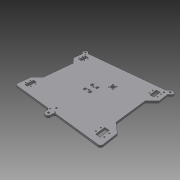
# Autodesk Inventor part: y_carriage_v2
Saved by Autodesk Inventor 2014 (Build 180170000, 170)
## iProperties
Created: 2013-12-03
Part Number: y_carriage_v2
Material: Generic
Document SubType Name: Modeling
Designer: buben
Density: 1 g/cm^3
Appearance: Default
Author: buben
Subject: Laser Cutted
Autodesk Inventor part; units mm, degrees
ref_plane "YZ Plane" through (0, 0, 0) normal (1, 0, 0) x (0, 1, 0)
ref_plane "XZ Plane" through (0, 0, 0) normal (0, 1, 0) x (-1, 0, 0)
ref_plane "XY Plane" through (0, 0, 0) normal (0, 0, 1) x (1, 0, 0)
sketch "Sketch1" plane through (0, 0, 0) normal (0, 0, 1) x (1, 0, 0)
  line L0 (267.8905, 0) -> (267.8905, 212.6863)
  line L1 (256.5768, 224) -> (11.3137, 224)
  line L2 (0, 212.6863) -> (0, 0)
  line L3 (0, 224) -> (267.8905, 224) construction
  line L4 (267.8905, 224) -> (133.9453, -8) construction
  line L5 (133.9453, -8) -> (0, 224) construction
  circle A0 centre (0, 224) radius 2.75
  circle A1 centre (133.9453, -8) radius 2.75
  circle A2 centre (267.8905, 224) radius 2.75
  circle A3 centre (0, 224) radius 5 construction
  circle A4 centre (267.8905, 224) radius 5 construction
  circle A5 centre (133.9453, -8) radius 5 construction
  line L6 (-2.8284, 232.4853) -> (-8.4853, 226.8284)
  line L7 (-8.4853, 226.8284) -> (-8.4853, 221.1716)
  line L8 (-2.8284, 232.4853) -> (2.8284, 232.4853)
  line L9 (2.8284, 232.4853) -> (11.3137, 224)
  line L10 (-8.4853, 221.1716) -> (0, 212.6863)
  line L11 (125.9453, 0) -> (125.9453, -12)
  line L12 (125.9453, -12) -> (129.9453, -16)
  line L13 (129.9453, -16) -> (137.9453, -16)
  line L14 (137.9453, -16) -> (141.9453, -12)
  line L15 (141.9453, -12) -> (141.9453, 0)
  line L16 (267.8905, 212.6863) -> (276.3758, 221.1716)
  line L17 (276.3758, 221.1716) -> (276.3758, 226.8284)
  line L18 (276.3758, 226.8284) -> (270.719, 232.4853)
  line L19 (270.719, 232.4853) -> (265.0621, 232.4853)
  line L20 (265.0621, 232.4853) -> (256.5768, 224)
  line L21 (0, 0) -> (125.9453, 0)
  line L22 (141.9453, 0) -> (267.8905, 0)
  dimension "d0" = 5.5
  dimension "d1" = 5.5
  dimension "d2" = 5.5
  dimension "d3" = 10
  dimension "d4" = 10
  dimension "d5" = 10
  dimension "d6" = 232
  dimension "d7" = 45
  dimension "d8" = 8
  dimension "d9" = 4
  dimension "d10" = 8
  dimension "d11" = 8
  dimension "d12" = 4
  dimension "d13" = 45
  dimension "d15" = 12
  dimension "d17" = 45
  dimension "d18" = 8
  dimension "d19" = 4
  dimension "d20" = 8
  dimension "d45" = 45
  dimension "d46" = 8
  dimension "d47" = 45
  dimension "d48" = 8
  dimension "d49" = 8
  dimension "d50" = 8
  constraints: 46 end point, 10 perpendicular, 7 coincident, 7 equal length, 6 centre point, 6 parallel, 2 collinear, 2 horizontal
  measures "d0" diameter of A1
  measures "d1" diameter of A0
  measures "d2" diameter of A2
  measures "d3" diameter of A4
  measures "d4" diameter of A5
  measures "d5" diameter of A3
  measures "d6" distance from line of L3 L4.end
  measures "d7" angle of L7 L6
  measures "d8" distance from line of L3.start L6
  measures "d9" distance from line of L6.end L10
  measures "d10" distance of L6.start L6.end
  measures "d11" distance of L12.end L13.end
  measures "d12" horizontal distance of L11.end L12.end
  measures "d13" angle of L13 L12
  measures "d15" distance of L14.end L15.end
  measures "d17" angle of L17 L18
  measures "d18" distance of L17.end L18.end
  measures "d19" distance from line of L18.end L20
  measures "d20" distance from line of L18 L3.end
  measures "d45" angle of L9 L1
  measures "d46" distance from line of L10 L3.start
  measures "d47" angle of L20 L1
  measures "d48" distance from line of L20 L3.end
  measures "d49" distance from line of L13 L4.end
  measures "d50" distance from line of L11 L4.end
extrude "Extrusion2" add sketch "Sketch1" along normal blind 6
sketch "Sketch3" plane through (0, 0, 6) normal (0, 0, 1) x (1, 0, 0)
  line L0 (0, 212.6863) -> (0, 0) projected
  line L1 (0, 0) -> (125.9453, 0) projected
  line L2 (267.8905, 0) -> (267.8905, 212.6863) projected
  line L3 (256.5768, 224) -> (11.3137, 224) projected
  line L4 (16.4453, 209) -> (25.4453, 209)
  line L5 (26.4453, 208) -> (26.4453, 185)
  line L6 (25.4453, 184) -> (16.4453, 184)
  line L7 (15.4453, 185) -> (15.4453, 208)
  arc A0 (16.4453, 209) -> (15.4453, 208) centre (16.4453, 208) ccw
  arc A1 (15.4453, 185) -> (16.4453, 184) centre (16.4453, 185) ccw
  arc A2 (25.4453, 184) -> (26.4453, 185) centre (25.4453, 185) ccw
  arc A3 (26.4453, 208) -> (25.4453, 209) centre (25.4453, 208) ccw
  line L8 (242.4453, 209) -> (251.4453, 209)
  line L9 (252.4453, 208) -> (252.4453, 185)
  line L10 (251.4453, 184) -> (242.4453, 184)
  line L11 (241.4453, 185) -> (241.4453, 208)
  arc A4 (242.4453, 209) -> (241.4453, 208) centre (242.4453, 208) ccw
  arc A5 (241.4453, 185) -> (242.4453, 184) centre (242.4453, 185) ccw
  arc A6 (251.4453, 184) -> (252.4453, 185) centre (251.4453, 185) ccw
  arc A7 (252.4453, 208) -> (251.4453, 209) centre (251.4453, 208) ccw
  line L12 (242.4453, 40) -> (251.4453, 40)
  line L13 (252.4453, 39) -> (252.4453, 16)
  line L14 (251.4453, 15) -> (242.4453, 15)
  line L15 (241.4453, 16) -> (241.4453, 39)
  arc A8 (242.4453, 40) -> (241.4453, 39) centre (242.4453, 39) ccw
  arc A9 (241.4453, 16) -> (242.4453, 15) centre (242.4453, 16) ccw
  arc A10 (251.4453, 15) -> (252.4453, 16) centre (251.4453, 16) ccw
  arc A11 (252.4453, 39) -> (251.4453, 40) centre (251.4453, 39) ccw
  line L16 (16.4453, 40) -> (25.4453, 40)
  line L17 (26.4453, 39) -> (26.4453, 16)
  line L18 (25.4453, 15) -> (16.4453, 15)
  line L19 (15.4453, 16) -> (15.4453, 39)
  arc A12 (16.4453, 40) -> (15.4453, 39) centre (16.4453, 39) ccw
  arc A13 (15.4453, 16) -> (16.4453, 15) centre (16.4453, 16) ccw
  arc A14 (25.4453, 15) -> (26.4453, 16) centre (25.4453, 16) ccw
  arc A15 (26.4453, 39) -> (25.4453, 40) centre (25.4453, 39) ccw
  line L20 (0, 180) -> (20.9453, 159.0547)
  line L21 (20.9453, 159.0547) -> (20.9453, 64.9453)
  line L22 (20.9453, 64.9453) -> (0, 44)
  line L23 (267.8905, 180) -> (246.9453, 159.0547)
  line L24 (246.9453, 159.0547) -> (246.9453, 64.9453)
  line L25 (246.9453, 64.9453) -> (267.8905, 44)
  line L26 (0, 180) -> (0, 44)
  line L27 (267.8905, 180) -> (267.8905, 44)
  line L28 (-8.4853, 226.8284) -> (-8.4853, 221.1716) projected
  line L29 (26.4453, 196.5) -> (241.4453, 196.5) construction
  point P0 (20.9453, 184)
  point P1 (20.9453, 40)
  point P2 (246.9453, 184)
  point P3 (246.9453, 40)
  point P4 (26.4453, 27.5)
  point P5 (241.4453, 27.5)
  point P6 (133.9453, 196.5)
  point P7 (133.9453, 224)
  dimension "d66" = 1
  dimension "d67" = 11
  dimension "d68" = 25
  dimension "d69" = 1
  dimension "d70" = 11
  dimension "d71" = 25
  dimension "d72" = 1
  dimension "d73" = 11
  dimension "d74" = 25
  dimension "d75" = 1
  dimension "d76" = 11
  dimension "d77" = 25
  dimension "d82" = 15
  dimension "d84" = 45
  dimension "d85" = 45
  dimension "d86" = 15
  dimension "d88" = 4
  dimension "d89" = 4
  dimension "d139" = 226
  constraints: 50 end point, 32 point on circle, 32 tangent, 16 centre point, 12 equal radius, 10 midpoint, 9 parallel, 8 perpendicular, 5 vertical alignment, 4 horizontal, 4 horizontal alignment, 4 point on line, 2 collinear
  measures "d66" radius of A0
  measures "d67" distance between parallel lines of L5 L7
  measures "d68" distance between parallel lines of L6 L4
  measures "d69" radius of A4
  measures "d70" distance between parallel lines of L9 L11
  measures "d71" distance between parallel lines of L10 L8
  measures "d72" radius of A8
  measures "d73" distance between parallel lines of L13 L15
  measures "d74" distance between parallel lines of L14 L12
  measures "d75" radius of A12
  measures "d76" distance between parallel lines of L17 L19
  measures "d77" distance between parallel lines of L18 L16
  measures "d82" distance between parallel lines of L3 L4
  measures "d84" angle of L2 L23
  measures "d85" angle of L0 L20
  measures "d86" distance between parallel lines of L1 L18
  measures "d88" distance from line of L22.end L16
  measures "d89" distance from line of L6 L20.start
  measures "d139" distance of point (246.945, 184) point (20.945, 184)
extrude "Extrusion3" cut sketch "Sketch3" against normal blind 6
chamfer "Chamfer1" distance 4 angle 45 4 edges at (0, 0, 3) (125.9453, 0, 3) (141.9453, 0, 3) (267.8905, 0, 3)
sketch "Sketch6" plane through (0, 0, 6) normal (0, 0, 1) x (1, 0, 0)
  line L0 (276.3758, 226.8284) -> (270.719, 232.4853) projected
  line L1 (-2.8284, 232.4853) -> (-8.4853, 226.8284) projected
  line L2 (16.4453, 40) -> (25.4453, 40) projected
  circle A0 centre (267.8905, 224) radius 2.75 projected
  circle A1 centre (133.9453, -8) radius 2.75 projected
  circle A2 centre (0, 224) radius 2.75 projected
  circle A3 centre (9.8995, 214.1005) radius 2.25
  line L3 (-5.6569, 229.6569) -> (9.8995, 214.1005) construction
  circle A4 centre (9.8995, 214.1005) radius 4.5 construction
  circle A5 centre (0, 224) radius 5 construction
  line L4 (11.3137, 224) -> (0, 212.6863) construction
  circle A6 centre (257.991, 214.1005) radius 2.25
  line L5 (273.5474, 229.6569) -> (257.991, 214.1005) construction
  circle A7 centre (133.9453, 12) radius 2.25
  circle A8 centre (125.9453, 2) radius 1.5
  circle A9 centre (141.9453, 2) radius 1.5
  line L6 (133.9453, -8) -> (133.9453, 12) construction
  circle A10 centre (133.9453, 12) radius 4.5 construction
  point P0 (125.9453, -4)
  point P1 (141.9453, -4)
  point P2 (0, 0)
  dimension "d103" = 4.5
  dimension "d105" = 14
  dimension "d106" = 10
  dimension "d107" = 9
  dimension "d108" = 4.5
  dimension "d109" = 14
  dimension "d110" = 4.5
  dimension "d111" = 20
  dimension "d112" = 3
  dimension "d113" = 9
  dimension "d114" = 10
  constraints: 8 centre point, 8 end point, 3 coincident, 3 vertical alignment, 2 midpoint, 2 perpendicular, 2 point on line, 1 equal radius, 1 horizontal alignment
  measures "d103" diameter of A3
  measures "d105" distance of L3.end A2.centre
  measures "d106" diameter of A5
  measures "d107" diameter of A4
  measures "d108" diameter of A6
  measures "d109" distance of L5.end A0.centre
  measures "d110" diameter of A7
  measures "d111" distance of L6.start L6.end
  measures "d112" diameter of A8
  measures "d113" diameter of A10
  measures "d114" vertical distance of L6.start A9.centre
extrude "Extrusion4" cut sketch "Sketch6" against normal through all contours A3 | A6 | A7 | A8 | A9
sketch "Sketch7" plane through (0, 0, 6) normal (0, 0, 1) x (1, 0, 0)
  line L0 (4, 0) -> (121.9453, 0) projected
  circle A0 centre (133.9453, -8) radius 2.75 projected
  line L1 (122.9453, 127.5) -> (128.9453, 127.5)
  line L2 (128.9453, 127.5) -> (128.9453, 119.5)
  line L3 (128.9453, 119.5) -> (122.9453, 119.5)
  line L4 (122.9453, 119.5) -> (122.9453, 127.5)
  line L5 (138.9453, 127.5) -> (144.9453, 127.5)
  line L6 (144.9453, 127.5) -> (144.9453, 119.5)
  line L7 (144.9453, 119.5) -> (138.9453, 119.5)
  line L8 (138.9453, 119.5) -> (138.9453, 127.5)
  line L9 (122.9453, 104.5) -> (128.9453, 104.5)
  line L10 (128.9453, 104.5) -> (128.9453, 96.5)
  line L11 (128.9453, 96.5) -> (122.9453, 96.5)
  line L12 (122.9453, 96.5) -> (122.9453, 104.5)
  line L13 (138.9453, 104.5) -> (144.9453, 104.5)
  line L14 (144.9453, 104.5) -> (144.9453, 96.5)
  line L15 (144.9453, 96.5) -> (138.9453, 96.5)
  line L16 (138.9453, 96.5) -> (138.9453, 104.5)
  line L17 (128.9453, 119.5) -> (138.9453, 104.5) construction
  line L18 (128.9453, 104.5) -> (138.9453, 119.5) construction
  circle A1 centre (133.9453, 119.5) radius 2.25
  circle A2 centre (133.9453, 104.5) radius 2.25
  line L19 (133.9453, 119.5) -> (133.9453, 104.5) construction
  point P0 (0, 0)
  point P1 (133.9453, 112)
  dimension "d117" = 6
  dimension "d118" = 8
  dimension "d119" = 8
  dimension "d120" = 6
  dimension "d121" = 112
  dimension "d122" = 10
  dimension "d123" = 15
  dimension "d124" = 4.5
  dimension "d125" = 15
  constraints: 38 end point, 8 collinear, 8 parallel, 4 horizontal, 4 perpendicular, 2 centre point, 2 midpoint, 2 vertical alignment, 1 coincident, 1 equal radius
  measures "d117" distance of L1.start L1.end
  measures "d118" distance of L3.end L1.start
  measures "d119" distance of L11.end L9.start
  measures "d120" distance of L5.start L5.end
  measures "d121" distance from line of point (133.945, 112) L0
  measures "d122" distance between parallel lines of L16 L10
  measures "d123" distance between parallel lines of L13 L7
  measures "d124" diameter of A1
  measures "d125" distance of L19.start L19.end
extrude "Extrusion5" cut sketch "Sketch7" against normal through all contours L1 L2 L3 L4 | L5 L6 L7 L8 | L9 L10 L11 L12 | L13 L14 L15 L16 | A1 | A2
sketch "Sketch8" plane through (0, 0, 6) normal (0, 0, 1) x (1, 0, 0)
  line L0 (15.4453, 185) -> (15.4453, 208) projected
  line L1 (16.4453, 209) -> (25.4453, 209) projected
  line L2 (26.4453, 208) -> (26.4453, 185) projected
  line L3 (25.4453, 184) -> (16.4453, 184) projected
  line L4 (252.4453, 208) -> (252.4453, 185) projected
  line L5 (241.4453, 185) -> (241.4453, 208) projected
  line L6 (25.4453, 15) -> (16.4453, 15) projected
  line L7 (16.4453, 40) -> (25.4453, 40) projected
  circle A0 centre (10.4453, 203) radius 1.5
  circle A1 centre (31.4453, 203) radius 1.5
  circle A2 centre (10.4453, 190) radius 1.5
  circle A3 centre (31.4453, 190) radius 1.5
  circle A4 centre (236.4453, 203) radius 1.5
  circle A5 centre (257.4453, 203) radius 1.5
  circle A6 centre (257.4453, 190) radius 1.5
  circle A7 centre (236.4453, 190) radius 1.5
  circle A8 centre (10.4453, 34) radius 1.5
  circle A9 centre (31.4453, 34) radius 1.5
  circle A10 centre (10.4453, 21) radius 1.5
  circle A11 centre (31.4453, 21) radius 1.5
  circle A12 centre (236.4453, 34) radius 1.5
  circle A13 centre (236.4453, 21) radius 1.5
  circle A14 centre (257.4453, 34) radius 1.5
  circle A15 centre (257.4453, 21) radius 1.5
  point P0 (0, 0)
  dimension "d128" = 3
  dimension "d129" = 6
  dimension "d130" = 6
  dimension "d131" = 5
  dimension "d132" = 5
  dimension "d133" = 6
  dimension "d134" = 6
  dimension "d135" = 5
  dimension "d136" = 5
  constraints: 16 centre point, 15 equal radius, 12 horizontal alignment, 12 vertical alignment
  measures "d128" diameter of A0
  measures "d129" distance from line of A0.centre L1
  measures "d130" distance from line of L3 A2.centre
  measures "d131" distance from line of A0.centre L0
  measures "d132" distance from line of L2 A1.centre
  measures "d133" distance from line of A8.centre L7
  measures "d134" distance from line of A10.centre L6
  measures "d135" distance from line of A4.centre L5
  measures "d136" distance from line of L4 A5.centre
extrude "Extrusion6" cut sketch "Sketch8" against normal through all
sketch "Sketch9" plane through (0, 0, 6) normal (0, 0, 1) x (1, 0, 0)
  line L0 (158.9453, 157.4853) -> (170.9453, 157.4853) construction
  line L1 (170.9453, 157.4853) -> (170.9453, 143.4853) construction
  line L2 (170.9453, 143.4853) -> (158.9453, 143.4853) construction
  line L3 (158.9453, 143.4853) -> (158.9453, 157.4853) construction
  circle A0 centre (158.9453, 143.4853) radius 1.6
  circle A1 centre (170.9453, 143.4853) radius 1.6
  circle A2 centre (170.9453, 157.4853) radius 1.6
  circle A3 centre (158.9453, 157.4853) radius 1.6
  line L4 (162.9453, 156.4853) -> (166.9453, 156.4853)
  line L5 (170.9453, 152.4853) -> (170.9453, 148.4853)
  line L6 (166.9453, 144.4853) -> (162.9453, 144.4853)
  line L7 (158.9453, 148.4853) -> (158.9453, 152.4853)
  line L8 (158.9453, 148.4853) -> (162.9453, 144.4853)
  line L9 (166.9453, 144.4853) -> (170.9453, 148.4853)
  line L10 (170.9453, 152.4853) -> (166.9453, 156.4853)
  line L11 (162.9453, 156.4853) -> (158.9453, 152.4853)
  line L12 (158.9453, 172.4853) -> (170.9453, 172.4853) construction
  line L13 (170.9453, 172.4853) -> (170.9453, 156.4853) construction
  line L14 (170.9453, 156.4853) -> (158.9453, 156.4853) construction
  line L15 (158.9453, 156.4853) -> (158.9453, 172.4853) construction
  line L16 (144.9453, 127.5) -> (144.9453, 119.5) projected
  line L17 (2.8284, 232.4853) -> (-2.8284, 232.4853) projected
  point P0 (0, 0)
  point P1 (164.9453, 156.4853)
  point P2 (164.9453, 157.4853)
  dimension "d140" = 3.2
  dimension "d141" = 14
  dimension "d142" = 12
  dimension "d143" = 45
  dimension "d144" = 4
  dimension "d145" = 1
  dimension "d146" = 4
  dimension "d148" = 16
  dimension "d152" = 60
  dimension "d153" = 14
  constraints: 32 end point, 10 perpendicular, 6 parallel, 4 centre point, 4 coincident, 3 collinear, 3 equal radius, 3 horizontal, 2 midpoint, 1 vertical alignment
  measures "d140" diameter of A0
  measures "d141" distance of L2.end L0.start
  measures "d142" distance of L0.start L0.end
  measures "d143" angle of L6 L8
  measures "d144" distance of L6.start L6.end
  measures "d145" distance between parallel lines of L4 L0
  measures "d146" horizontal distance of L6.end L7.start
  measures "d148" distance of L14.end L12.start
  measures "d152" distance between parallel lines of L17 L12
  measures "d153" distance from line of A0.centre L16
extrude "Extrusion7" cut sketch "Sketch9" against normal through all
body "Solid2"
